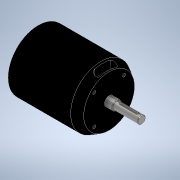
# Autodesk Inventor part: Flipsky 6374
Saved by Autodesk Inventor 2021 (Build 250183000, 183)
## iProperties
Created: 2020-09-11
Part Number: Flipsky 6374
Material: Aluminum 6061
Document SubType Name: Modeling
Designer: sami8
Density: 2.7 g/cm^3
Appearance: Aluminum - Flat
Author: sami8
Autodesk Inventor part; units mm, degrees
ref_plane "YZ Plane" through (0, 0, 0) normal (1, 0, 0) x (0, 1, 0)
ref_plane "XY Plane" through (0, 0, 0) normal (0, 0, 1) x (1, 0, 0)
sketch "Sketch1" plane through (0, 0, 0) normal (1, 0, 0) x (0, 1, 0)
  circle A0 centre (0, 0) radius 31.5
  circle A1 centre (0, 0) radius 5
  circle A2 centre (0, 0) radius 4
  circle A3 centre (0, 0) radius 22 construction
  circle A4 centre (15.5563, -15.5563) radius 2
  line L0 (0, 0) -> (15.5563, -15.5563) construction
  line L1 (0, 0) -> (22, 0) construction
  circle A5 centre (15.5563, 15.5563) radius 2
  circle A6 centre (-15.5563, 15.5563) radius 2
  circle A7 centre (-15.5563, -15.5563) radius 2
  dimension "d0" = 63
  dimension "d1" = 10
  dimension "d2" = 8
  dimension "d3" = 44
  dimension "d4" = 4
  dimension "d33" = 45
  dimension "d36" = 360
  constraints: 8 centre point, 4 coincident, 4 end point, 2 point on circle, 1 horizontal, 9 other
  measures "d0" diameter of A0
  measures "d1" diameter of A1
  measures "d2" diameter of A2
  measures "d3" diameter of A3
  measures "d4" diameter of A4
  measures "d33" angle of L0 L1
extrude "Extrusion1" add sketch "Sketch1" against normal blind 74 contours A0 | A4 | A5 | A6 | A7
extrude "Extrusion2" add sketch "Sketch1" along normal blind 8 and the other way blind 74 separate body contours A1 | A2
extrude "Extrusion3" add sketch "Sketch1" along normal blind 34 contours A2 bodies 2
ref_plane "Work Plane1" through (0, 4, 0) normal (0, 1, 0) x (-1, 0, 0)
sketch "Sketch2" plane through (0, 4, 0) normal (0, 1, 0) x (-1, 0, 0)
  line L0 (-34, 4) -> (-34, -4) projected
  line L1 (-34, 0) -> (-8, 0) construction
  line L2 (-8, 5) -> (-8, -5) projected
  line L3 (-29.5, 0) -> (-12.5, 0) construction
  line L4 (-29.5, -1.5) -> (-12.5, -1.5)
  line L5 (-12.5, 1.5) -> (-29.5, 1.5)
  arc A0 (-29.5, 1.5) -> (-29.5, -1.5) centre (-29.5, 0) ccw
  arc A1 (-12.5, -1.5) -> (-12.5, 1.5) centre (-12.5, 0) ccw
  line L6 (-21, 0) -> (-4, 0) construction
  point P0 (0, 0)
  dimension "d25" = 8.5
  dimension "d26" = 0
  dimension "d27" = 3
  constraints: 12 end point, 4 midpoint, 4 point on circle, 4 tangent, 2 centre point, 2 collinear, 1 horizontal, 1 parallel
  measures "d25" distance of L6.start L3.end
  measures "d26" distance between parallel lines of L3 L6
  measures "d27" diameter of A1
extrude "Extrusion4" cut sketch "Sketch2" against normal blind 2 bodies 2
ref_plane "Work Plane2" through (0, 31.5, 0) normal (0, 1, 0) x (-1, 0, 0)
sketch "Sketch3" plane through (0, 31.5, 0) normal (0, 1, 0) x (-1, 0, 0)
  line L0 (0, 0) -> (4, 0) construction
  line L1 (4, 8) -> (4, -8) construction
  line L2 (1, 8) -> (1, -8)
  line L3 (7, -8) -> (7, 8)
  arc A0 (7, 8) -> (1, 8) centre (4, 8) ccw
  arc A1 (1, -8) -> (7, -8) centre (4, -8) ccw
  dimension "d38" = 4
  dimension "d39" = 8
  dimension "d40" = 6
  constraints: 10 end point, 4 point on circle, 4 tangent, 2 centre point, 1 horizontal, 1 midpoint, 1 parallel, 1 vertical
  measures "d38" distance of L0.start L0.end
  measures "d39" distance of L0.end L1.end
  measures "d40" diameter of A1
extrude "Extrusion5" cut sketch "Sketch3" against normal blind 10 bodies 1
hole "Hole1" at (0, 15.5563, -15.5563) at (0, 15.5563, 15.5563) at (0, -15.5563, 15.5563) at (0, -15.5563, -15.5563) direction (-1, 0, 0) diameter 3.242 depth 5 tip angle 118 bodies 1 thread size "M4x0.7" class "6H" standard "ANSI Metric M Profile"
chamfer "Chamfer1" distance 5 angle 60 1 edges at (0, -31.5, 0) measured on face at (0, -31, 0)
chamfer "Chamfer2" distance 0.5 angle 45 2 edges at (34, -4, 0) (8, -5, 0)
body "Solid1"
body "Solid2"
